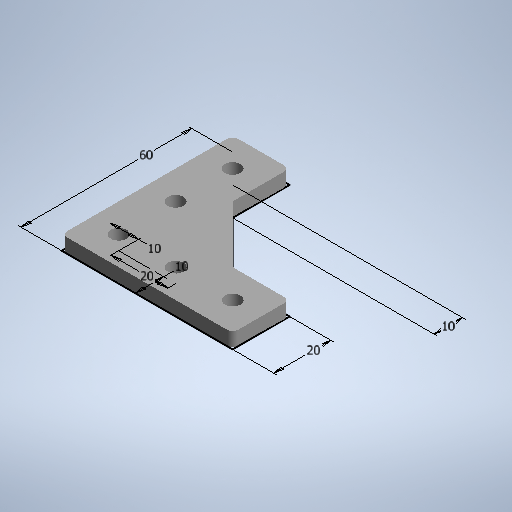
# Autodesk Inventor part: 6060L
Saved by Autodesk Inventor 2025.4 (Build 294407000, 407)
## iProperties
Created: 2026-07-08
Part Number: 6060L
Material: Générique
Document SubType Name: Modeling
Designer: louis
Density: 1 g/cm^3
Appearance: Par défaut
Author: louis
Autodesk Inventor part; units mm, degrees
ref_plane "YZ Plane" through (0, 0, 0) normal (1, 0, 0) x (0, 1, 0)
ref_plane "XZ Plane" through (0, 0, 0) normal (0, 1, 0) x (-1, 0, 0)
ref_plane "XY Plane" through (0, 0, 0) normal (0, 0, 1) x (1, 0, 0)
sketch "Sketch2" plane through (0, 0, 0) normal (0, 0, 1) x (1, 0, 0)
  line L0 (0, 0) -> (0, 20) construction
  line L1 (0, 20) -> (0, 40) construction
  line L2 (0, 0) -> (20, 0) construction
  line L3 (20, 0) -> (40, 0) construction
  line L4 (-10, -10) -> (-10, 50)
  line L5 (-10, 50) -> (10, 50)
  line L6 (10, 50) -> (10, 30)
  line L7 (10, 30) -> (30, 10)
  line L8 (30, 10) -> (50, 10)
  line L9 (50, 10) -> (50, -10)
  line L10 (50, -10) -> (-10, -10)
  dimension "d0" = 20
  dimension "d1" = 20
  dimension "d2" = 60
  dimension "d3" = 10
  dimension "d4" = 10
  dimension "d5" = 10
  constraints: 22 end point, 6 equal length, 5 coincident, 4 horizontal, 2 perpendicular, 2 point on line, 1 parallel, 1 vertical
  measures "d0" distance of L0.start L2.end
  measures "d1" distance of L8.end L9.end
  measures "d2" distance of L4.start L4.end
  measures "d3" distance from line of L0.start L4
  measures "d4" distance from line of L10 L0.start
  measures "d5" horizontal distance of L1.end L6.end
extrude "Extrusion1" add sketch "Sketch2" along normal blind 5
hole "Hole1" at (0, 40, 0) at (0, 20, 0) at (20, 0, 0) at (40, 0, 0) at (0, 0, 0) direction (0, 0, 1) diameter 5.5 end through all clearance for "Flat Head Machine Screw" size "M5" standard "Ansi Metric M Profile"
fillet "Fillet1" radius 2 7 edges at (-10, 50, 2.5) (10, 50, 2.5) (10, 30, 2.5) (-10, -10, 2.5) (30, 10, 2.5) (50, 10, 2.5) (50, -10, 2.5)
body "Solid1"
